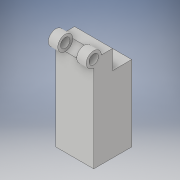
# Autodesk Inventor part: upper leg
Saved by Autodesk Inventor 2019 (Build 230136000, 136)
## iProperties
Created: 2018-07-06
Part Number: upper leg
Material: Generic
Document SubType Name: Modeling
Designer: HIVE
Density: 1 g/cm^3
Appearance: Default
Author: HIVE
Autodesk Inventor part; units mm, degrees
ref_plane "YZ Plane" through (0, 0, 0) normal (1, 0, 0) x (0, 1, 0)
ref_plane "XZ Plane" through (0, 0, 0) normal (0, 1, 0) x (-1, 0, 0)
ref_plane "XY Plane" through (0, 0, 0) normal (0, 0, 1) x (1, 0, 0)
sketch "Sketch1" plane through (0, 0, 0) normal (0, 1, 0) x (-1, 0, 0)
  line L0 (0, 0) -> (40, 0)
  line L1 (40, 0) -> (40, -40)
  line L2 (40, -40) -> (0, -40)
  line L3 (0, -40) -> (0, 0)
  dimension "d2" = 40
  dimension "d3" = 40
  constraints: 8 end point, 2 parallel, 1 horizontal, 1 perpendicular
  measures "d2" distance of L1.end L2.end
  measures "d3" distance of L0.end L1.end
extrude "Extrusion1" add sketch "Sketch1" along normal blind 100
ref_plane "Work Plane1" through (-20, 0, 0) normal (1, 0, 0) x (0, 0, -1)
sketch "Sketch2" plane through (-20, 0, 0) normal (1, 0, 0) x (0, 0, -1)
  line L0 (40, 0) -> (0, 0) projected
  line L1 (40, 0) -> (40, 100) projected
  line L2 (0, 100) -> (40, 100) projected
  line L3 (0, 0) -> (0, 100) projected
  circle A0 centre (0, 100) radius 5
  line L4 (40, 100) -> (0, 100) projected
  circle A1 centre (0, 100) radius 7.9
  dimension "d4" = 15.8
  dimension "d5" = 10
  constraints: 2 centre point, 2 coincident
  measures "d4" diameter of A1
  measures "d5" diameter of A0
extrude "Extrusion2" add sketch "Sketch2" along normal mid plane 40 contours A1 L2 A0 L3 | L3 A0 L2 A1
extrude "Extrusion3" cut sketch "Sketch2" along normal mid plane 40 contours A0 L2 L3 | L3 L2 A0
extrude "Extrusion4" cut sketch "Sketch2" along normal mid plane 20 contours A1 L2 A0 L3 | L3 A0 L2 A1
sketch "Sketch3" plane through (0, 0, 0) normal (1, 0, 0) x (0, 0, -1)
  line L0 (40, 100) -> (19.8, 100)
  line L1 (19.8, 100) -> (19.8, 79.8)
  line L2 (19.8, 79.8) -> (40, 79.8)
  line L3 (40, 79.8) -> (40, 100)
  point P0 (0, 0)
  dimension "d12" = 20.2
  dimension "d13" = 20.2
  constraints: 8 end point, 2 parallel, 1 horizontal, 1 perpendicular
  measures "d12" distance of L2.end L1.end
  measures "d13" distance of L0.end L1.end
extrude "Extrusion5" cut sketch "Sketch3" against normal through all
equation "\"d2\" = legDiam"
equation "\"d3\" = legDiam"
equation "\"d5\" = hingeHoleDiam"
equation "\"d6\" = legDiam"
equation "\"d8\" = legDiam"
equation "\"d10\" = 0.5 * legDiam"
equation "\"d12\" = kneeBallDepth + clearance"
equation "\"d13\" = kneeBallLocationExtend + kneeBallLocationUp + clearance"
equation "\"legDiam\" = 40"
equation "\"hingeHoleDiam\" = 10"
equation "\"kneeBallDepth\" = 20"
equation "\"clearance\" = 0.2"
equation "\"kneeBallLocationExtend\" = 10"
equation "\"kneeBallLocationUp\" = 10"
body "Solid1"
